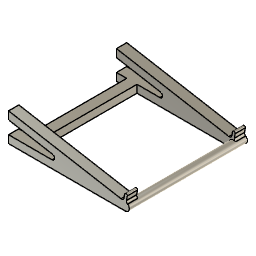
Laptop_Stand (Autodesk Fusion 360 design; units mm, degrees)
Autodesk Fusion 360 part; units mm, degrees
note: some values were not read from the file. Chosen so that the rebuilt part matches the saved one: a direction; which face or edge a step refers to.
sketch "Sketch1" plane through (0, 0, 0) normal (0, 0, 1) x (1, 0, 0)
  line L0 (-227.5, 7.5) -> (-227.5, -7.5)
  line L1 (-227.5, -7.5) -> (0, -7.5)
  line L2 (-227.5, 7.5) -> (0, 7.5)
  arc A0 (-0.039698, 7.5) -> (-0.039698, -7.5) centre (-0.039698, 0) cw
  dimension "d8" = 227.5
  dimension "d9" = 7.5
  constraint perpendicular L0 L1
  constraint perpendicular L0 L2
  constraint tangent L1 A0
  constraint tangent L2 A0
  measures "d8" distance of origin L0
  measures "d9" radius of A0
sketch "Sketch2" plane through (0, 0, 0) normal (0, 0, 1) x (1, 0, 0)
  line L0 (-1.302361, -7.386058) -> (-227.5, 32.498689)
  line L1 (-224.895277, 47.270805) -> (1.302361, 7.386058)
  line L2 (-224.895277, 47.270805) -> (-227.5, 47.730088)
  line L3 (-227.5, 47.730088) -> (-227.5, 32.498689)
  arc A0 (-1.302361, -7.386058) -> (1.302361, 7.386058) centre (0, 0) ccw
  line L4 (-227.5, 32.498689) -> (-224.895277, 47.270805) construction
  line L5 (0, 0) -> (-226.197639, 39.884747) construction
  line L6 (0, 0) -> (-3.591174, 0) construction
  line L7 (-227.5, 7.5) -> (-227.5, -7.5)
  dimension "d22" = 10
  dimension "d23" = 7.5
  constraint coincident A0.centre L5.start
  constraint tangent L0 A0
  constraint tangent L1 A0
  constraint perpendicular L1 L4
  constraint perpendicular L0 L4
  constraint horizontal L6
  constraint vertical L3
  constraint collinear L3 L7
  constraint collinear L1 L2
  measures "d22" angle of L5 L6
  measures "d23" radius of A0
extrude "Extrude2" add sketch "Sketch1" sketch "Sketch2" along normal mid plane 20 contours L0 L1 L2 A0 picked at (-75.859799, -2.5) of sketch 2 contours L0 L1 L2 L3 A0 picked at (-75.833333, 10.832896) makes body 1
sketch "Sketch3" plane through (1.302361, 7.386058, 0) normal (0.173648, 0.984808, 0) x (-0.984808, 0.173648, 0)
  line L0 (232.332007, -10) -> (232.332007, 10)
  line L1 (232.332007, 10) -> (0, 10)
  line L2 (0, 10) -> (0, -10)
  line L3 (0, -10) -> (232.332007, -10)
  line L4 (0, 10) -> (5, 10)
  line L5 (5, 10) -> (5, -10)
  line L6 (5, -10) -> (0, -10)
  line L7 (0, -10) -> (0, 10)
  dimension "d27" = 5
  dimension "d28" = 20
  constraint horizontal L4
  constraint vertical L5
  constraint horizontal L6
  constraint vertical L7
  constraint coincident L1.end L2.start
  measures "d27" distance of L1.end L4.end
  measures "d28" distance of L1.end L2.end
extrude "Extrude3" add sketch "Sketch3" along normal blind 15 contours L1 L2 L3 L4 L5 L6 L7 picked at (1.666667, -3.333333) bodies 1
fillet "Fillet1" radius 2.5 2 edges at (-1.016955, 23.026415, 0) (3.907084, 22.158174, 0) on bodies 1
fillet "Fillet2" radius 5 2 edges at (1.302361, 7.386058, 5) (1.302361, 7.386058, -5) on bodies 1
fillet "Fillet3" radius 5 1 edges at (-3.621677, 8.254299, 0) on bodies 1
fillet "Fillet4" radius 5 2 edges at (-85.725392, 7.5, -5) (-85.725392, 7.5, 5) on bodies 1
copy_body "Body->Comp1" bodies 1 removing the originals makes body 2 in component "Leg"
move_body "Move1" bodies 2 to x (1, 0, 0) y (0, 0, 1) z (0, -1, 0) at (0, 0, 10) in component "Leg"
copy_body "CopyPasteBodies1" bodies 2 makes body 3 in component "Leg"
move_body "Move2" bodies 3 to x (1, 0, 0) y (0, 1, 0) z (0, 0, 1) at (0, 210, 0) in component "Leg"
sketch "Sketch1 (2)" plane through (0, 10, 0) normal (0, 1, 0) x (-1, 0, 0) in component "Leg"
  arc A0 (1.451075, 30.564396) -> (-3.472964, 29.696155) centre (-1.010944, 30.130276) ccw
  line L0 (-3.472964, 29.696155) -> (-1.98939, 21.28239)
  arc A1 (-4.148057, 16.24849) -> (-1.98939, 21.28239) centre (-6.913429, 20.414149) ccw
  arc A2 (-4.148057, 16.24849) -> (0.019849, 2.500026) centre (0, 10) ccw
  arc A3 (0.019849, 2.500026) -> (0.039698, 2.5) centre (0.039698, 10) ccw
  line L1 (0.039698, 2.5) -> (227.5, 2.5)
  line L2 (227.5, 2.5) -> (227.5, 17.5)
  line L3 (227.5, 17.5) -> (142.875653, 17.5)
  arc A4 (142.007412, 27.424039) -> (142.875653, 17.5) centre (142.875653, 22.5) ccw
  line L4 (142.007412, 27.424039) -> (227.5, 42.498689)
  line L5 (227.5, 42.498689) -> (227.5, 57.730088)
  line L6 (227.5, 57.730088) -> (8.545716, 19.12254)
  arc A5 (2.753437, 23.178338) -> (8.545716, 19.12254) centre (7.677475, 24.046579) ccw
  line L7 (2.753437, 23.178338) -> (1.451075, 30.564396)
  circle A6 centre (0, 10) radius 7.5
  dimension "d45" = 15
  constraint concentric A2 A6
  measures "d45" diameter of A6
extrude "Extrude1" add sketch "Sketch1 (2)" along normal blind 190 contours A2 A3 A6 picked at (3.176288, 7.286123) bodies 2 3 in component "Leg"
sketch "Sketch2 (2)" plane through (0, 10, 0) normal (0, 1, 0) x (-1, 0, 0) in component "Leg"
  arc A0 (0.019849, 2.500026) -> (-4.148057, 16.24849) centre (0, 10) ccw
  line L0 (0.039698, 2.5) -> (227.5, 2.5)
  line L1 (227.5, 2.5) -> (227.5, 17.5)
  line L2 (227.5, 17.5) -> (142.875653, 17.5)
  arc A1 (142.007412, 27.424039) -> (142.875653, 17.5) centre (142.875653, 22.5) ccw
  line L3 (142.007412, 27.424039) -> (227.5, 42.498689)
  line L4 (227.5, 42.498689) -> (227.5, 57.730088)
  line L5 (227.5, 57.730088) -> (8.545716, 19.12254)
  arc A2 (2.753437, 23.178338) -> (8.545716, 19.12254) centre (7.677475, 24.046579) ccw
  line L6 (2.753437, 23.178338) -> (1.451075, 30.564396)
  arc A3 (1.451075, 30.564396) -> (-3.472964, 29.696155) centre (-1.010944, 30.130276) ccw
  line L7 (-3.472964, 29.696155) -> (-1.98939, 21.28239)
  arc A4 (-4.148057, 16.24849) -> (-1.98939, 21.28239) centre (-6.913429, 20.414149) ccw
  line L8 (187.5, 17.5) -> (207.5, 17.5)
  line L9 (207.5, 17.5) -> (207.5, 2.5)
  line L10 (207.5, 2.5) -> (187.5, 2.5)
  line L11 (187.5, 2.5) -> (187.5, 17.5)
  arc A5 (0.019849, 2.500026) -> (0.039698, 2.5) centre (0.039698, 10) ccw
  dimension "d41" = 20
  dimension "d42" = 20
  constraint horizontal L8
  constraint vertical L9
  constraint horizontal L10
  constraint vertical L11
  constraint coincident L0 L9.end
  constraint coincident L2 L8.start
  measures "d41" distance of L1 L9
  measures "d42" distance of L9.end L10.end
extrude "Extrude2'" add sketch "Sketch2 (2)" along normal blind 190 contours L0 L2 L8 L9 L10 L11 picked at (194.166667, 12.5) bodies 2 in component "Leg"
component "Leg" placed x (1, 0, 0) y (0, 1, 0) z (0, 0, 1) at (0, 0, 0)
equation "Thickness = 15 mm"
equation "BaseLength = 235 mm"
equation "Width = 20 mm"
equation "d8 = BaseLength - ( Thickness / 2 )"
equation "d9 = Thickness / 2"
equation "TopAngle = 10 deg"
equation "TopLength = BaseLength / cos(TopAngle)"
equation "d22 = TopAngle"
equation "d23 = Thickness / 2"
equation "d24 = Width / 2"
equation "EndCapThickness = 5 mm"
equation "d27 = EndCapThickness"
equation "d28 = Width"
equation "EndCapHeight = 15 mm"
equation "d30 = EndCapHeight"
equation "StandWidth = 230 mm"
equation "d41 = Width"
equation "d42 = Width"
equation "d45 = Thickness"
